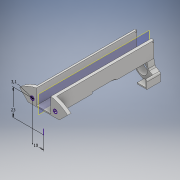
# Autodesk Inventor part: Hull_batt_pillar3
Saved by Autodesk Inventor 2018.2 (Build 222227000, 227)
## iProperties
Created: 2018-05-01
Part Number: Hull_batt_pillar3
Material: Generic
Document SubType Name: Modeling
Designer: suchanek
Density: 1 g/cm^3
Appearance: Default
Author: suchanek
Autodesk Inventor part; units mm, degrees
ref_plane "YZ Plane" through (0, 0, 0) normal (1, 0, 0) x (0, 1, 0)
ref_plane "XZ Plane" through (0, 0, 0) normal (0, 1, 0) x (-1, 0, 0)
ref_plane "XY Plane" through (0, 0, 0) normal (0, 0, 1) x (1, 0, 0)
sketch "Sketch1" plane through (0, 0, 0) normal (0, 1, 0) x (-1, 0, 0)
  arc A0 (21.0006, 25.4554) -> (6.35, 32.3833) centre (0, 0) ccw
  line L0 (0, 0) -> (-23.3345, 23.3345)
  line L1 (0, 0) -> (33, 0) construction
  line L2 (0, 0) -> (0, 8.3369)
  line L3 (-23.3345, 23.3345) -> (-9.1924, 9.1924)
  line L4 (-9.1924, 9.1924) -> (-6.965, 11.4198)
  line L5 (-6.965, 11.4198) -> (-13.7089, 18.1636)
  line L6 (-21.1071, 25.5619) -> (-23.3345, 23.3345)
  line L7 (23.3345, 23.3345) -> (9.1924, 9.1924)
  line L8 (9.1924, 9.1924) -> (6.965, 11.4198)
  line L9 (6.965, 11.4198) -> (13.7089, 18.1636)
  line L10 (21.1071, 25.5619) -> (23.3345, 23.3345)
  line L11 (-6.35, 32.3833) -> (6.35, 32.3833)
  line L12 (6.35, 32.3833) -> (6.35, 19.1636)
  line L13 (6.35, 19.1636) -> (-6.35, 19.1636)
  line L14 (-6.35, 19.1636) -> (-6.35, 32.3833)
  line L15 (13.7089, 18.1636) -> (-13.7089, 18.1636)
  line L16 (-13.7089, 18.1636) -> (-21.1071, 25.5619)
  arc A1 (-6.35, 32.3833) -> (-21.0006, 25.4554) centre (0, 0) ccw
  arc A2 (6.35, 32.3833) -> (-6.35, 32.3833) centre (0, 0) ccw
  line L17 (13.7089, 18.1636) -> (21.1071, 25.5619)
  point P0 (-6.35, 31.3636)
  dimension "d0" = 33
  dimension "d1" = 33
  dimension "d2" = 135
  dimension "d3" = 3.15
  dimension "d4" = 20
  dimension "d5" = 32
  dimension "d7" = 12.2
  dimension "d8" = 12.7
  dimension "d33" = 18.1636
  constraints: 36 end point, 7 point on circle, 6 point on line, 5 parallel, 4 symmetric about line, 3 centre point, 3 horizontal, 2 perpendicular, 1 coincident, 1 equal length, 1 vertical
  measures "d0" radius of A0
  measures "d1" distance of L0.start L0.end
  measures "d2" angle of L1 L0
  measures "d3" distance of L4.end L3.end
  measures "d4" distance between parallel lines of L6 L4
  measures "d5" distance of point (0, 0) point (-6.35, 31.364)
  measures "d7" distance of L13.end point (-6.35, 31.364)
  measures "d8" distance of L12.end L13.end
  measures "d33" distance from line of L0.start L15
extrude "Extrusion1" add sketch "Sketch1" along normal blind 3 contours L17 L15 L16 A1 L14 L13 L12 A0
sketch "Sketch2" plane through (0, 3, 0) normal (0, 1, 0) x (1, 0, 0)
  arc A0 (6.35, -32.3833) -> (21.0006, -25.4554) centre (0, 0) ccw projected
  line L0 (8.35, -31.9261) -> (8.35, -18.1636)
  line L1 (13.7089, -18.1636) -> (-13.7089, -18.1636) projected
  line L2 (-8.35, -18.1636) -> (-8.35, -31.9261)
  arc A1 (-21.0006, -25.4554) -> (-6.35, -32.3833) centre (0, 0) ccw projected
  line L3 (-6.35, -19.1636) -> (6.35, -19.1636) projected
  line L4 (6.35, -32.3833) -> (6.35, -19.1636)
  line L5 (6.35, -19.1636) -> (-6.35, -19.1636)
  line L6 (-6.35, -32.3833) -> (-6.35, -19.1636) projected
  line L7 (-6.35, -19.1636) -> (-6.35, -32.3833)
  dimension "d14" = 2
  constraints: 10 end point, 3 vertical, 2 perpendicular, 2 point on circle, 2 point on line, 1 horizontal alignment
  measures "d14" distance between parallel lines of L6 L2
extrude "Extrusion2" add sketch "Sketch2" along normal blind 85
ref_plane "Work Plane1" through (8.35, 3, 18.1636) normal (-0.7071068, 0, -0.7071068) x (0, 1, 0)
sketch "Sketch4" plane through (8.35, 3, 18.1636) normal (-0.7071068, 0, -0.7071068) x (0, 1, 0)
  circle A0 centre (49, 6.9393) radius 8
  line L0 (85, -9.7316) -> (85, 0) projected
  line L1 (-3, 3.7893) -> (0, 3.7893) projected
  line L2 (49, -1.0607) -> (31, -1.0607)
  line L3 (31, -1.0607) -> (31, 14.9393)
  line L4 (31, 14.9393) -> (49, 14.9393)
  line L5 (49, 14.9393) -> (49, -1.0607)
  point P0 (-3, 6.9393)
  dimension "d19" = 16
  dimension "d20" = 36
  dimension "d21" = 3.15
  dimension "d22" = 18
  dimension "d23" = 16
  constraints: 8 end point, 2 parallel, 2 point on circle, 1 centre point, 1 horizontal, 1 perpendicular
  measures "d19" diameter of A0
  measures "d20" distance from line of L0 A0.centre
  measures "d21" distance from line of L1 A0.centre
  measures "d22" distance of L3.end L4.end
  measures "d23" distance of L2.end L3.end
extrude "Extrusion3" cut sketch "Sketch4" along normal through all both and the other way through all
ref_plane "Work Plane3" through (0, 88, 18.1636) normal (-1, 0, 0) x (0, 0, 1)
mirror "Mirror1" about plane through (0, 88, 18.1636) normal (-1, 0, 0) of "Extrusion3"
sketch "Sketch5" plane through (0, 88, 0) normal (0, 1, 0) x (1, 0, 0)
  line L0 (8.35, -30.3833) -> (-8.35, -30.3833)
  line L1 (-8.35, -30.3833) -> (-8.35, -31.3833)
  line L2 (-8.35, -31.3833) -> (8.35, -31.3833)
  line L3 (8.35, -31.3833) -> (8.35, -30.3833)
  line L4 (8.35, -31.9261) -> (8.35, -18.1636) projected
  arc A0 (6.35, -32.3833) -> (21.0006, -25.4554) centre (0, 0) ccw projected
  dimension "d27" = 16.7
  dimension "d28" = 1
  dimension "d29" = 1
  constraints: 8 end point, 2 parallel, 1 collinear, 1 horizontal, 1 perpendicular
  measures "d27" distance of L2.end L1.end
  measures "d28" distance of L1.end L0.end
  measures "d29" distance from line of A0.start L2
extrude "Extrusion4" cut sketch "Sketch5" against normal blind 1.1
fillet "Fillet1" radius 0.5 4 edges at (7.35, 86.9, 31.3833) (-7.35, 86.9, 31.3833) (-7.35, 86.9, 30.3833) (7.35, 86.9, 30.3833)
sketch "Sketch6" plane through (13.7089, 0, 18.1636) normal (0, 0, -1) x (-1, 0, 0)
  line L0 (8.4589, 16) -> (18.9589, 16)
  line L1 (18.9589, 16) -> (18.9589, 54)
  line L2 (18.9589, 54) -> (8.4589, 54)
  line L3 (8.4589, 54) -> (8.4589, 16)
  line L4 (13.7089, 0) -> (13.7089, 8.6013)
  line L5 (5.3589, 88) -> (22.0589, 88) projected
  dimension "d36" = 10.5
  dimension "d37" = 38
  dimension "d38" = 34
  constraints: 10 end point, 2 parallel, 1 horizontal, 1 perpendicular, 1 vertical, 1 other
  measures "d36" distance of L1.end L2.end
  measures "d37" distance of L0.end L1.end
  measures "d38" distance between parallel lines of L5 L2
extrude "Extrusion5" cut sketch "Sketch6" against normal blind 0.336
sketch "Náčrt7" plane through (0, 0, 0) normal (0, -1, 0) x (1, 0, 0)
  circle A0 centre (-10, 23) radius 1.55
  line L0 (0, 0) -> (0, 4.6263)
  circle A1 centre (10, 23) radius 1.55
  dimension "d39" = 23
  dimension "d40" = 10
  dimension "d41" = 3.1
  constraints: 2 centre point, 2 end point, 1 symmetric about line, 1 vertical, 1 other
  measures "d39" vertical distance of L0.start A0.centre
  measures "d40" horizontal distance of L0.start A0.centre
  measures "d41" diameter of A0
extrude "Vysunutí6" cut sketch "Náčrt7" against normal up to surface (3 mm away)
sketch "Náčrt8" plane through (0, 0, 0) normal (0, -1, 0) x (1, 0, 0)
  line L0 (-10, 20.1132) -> (-12.5, 21.5566)
  line L1 (-12.5, 21.5566) -> (-12.5, 24.4434)
  line L2 (-12.5, 24.4434) -> (-10, 25.8868)
  line L3 (-10, 25.8868) -> (-7.5, 24.4434)
  line L4 (-7.5, 24.4434) -> (-7.5, 21.5566)
  line L5 (-7.5, 21.5566) -> (-10, 20.1132)
  point P0 (0, 0)
  point P1 (-10, 23)
  point P2 (-10, 23)
  dimension "d44" = 2.5
  constraints: 12 end point, 1 coincident, 13 other
  measures "d44" distance from line of L4 point (-10, 23)
extrude "Vysunutí7" cut sketch "Náčrt8" against normal blind 2 from surface at -3
ref_plane "Pracovní rovina4" through (0, 0, 19.1636) normal (-1, 0, 0) x (0, 0, 1)
mirror "Zrcadlit2" about plane through (0, 0, 19.1636) normal (-1, 0, 0) of "Vysunutí7"
sketch "Náčrt9" plane through (13.7089, 0, 18.4996) normal (0, 0, -1) x (-1, 0, 0)
  line L0 (15.4589, 47.589) -> (13.4589, 47.589)
  line L1 (13.4589, 47.589) -> (13.4589, 53.589)
  line L2 (13.4589, 53.589) -> (15.4589, 53.589)
  line L3 (15.4589, 53.589) -> (15.4589, 47.589)
  line L4 (15.4589, 17.089) -> (13.4589, 17.089)
  line L5 (13.4589, 17.089) -> (13.4589, 23.089)
  line L6 (13.4589, 23.089) -> (15.4589, 23.089)
  line L7 (15.4589, 23.089) -> (15.4589, 17.089)
  line L8 (5.3589, 88) -> (22.0589, 88) projected
  line L9 (13.7089, 105.6) -> (13.7089, -17.6) projected
  point P0 (13.7089, 0)
  dimension "d47" = 34.411
  dimension "d48" = 6
  dimension "d49" = 2
  dimension "d50" = 1.75
  dimension "d51" = 6
  dimension "d52" = 2
  dimension "d53" = 30.5
  constraints: 16 end point, 4 parallel, 2 horizontal, 2 perpendicular, 2 point on line
  measures "d47" distance between parallel lines of L2 L8
  measures "d48" distance between parallel lines of L0 L2
  measures "d49" distance between parallel lines of L1 L3
  measures "d50" distance between parallel lines of L9 L3
  measures "d51" distance between parallel lines of L4 L6
  measures "d52" distance of L5.end L6.end
  measures "d53" distance between parallel lines of L6 L2
extrude "Vysunutí8" add sketch "Náčrt9" along normal blind 5.5
sketch "Náčrt10" plane through (0.25, 17.089, 18.4996) normal (1, 0, 0) x (0, 0, -1)
  circle A0 centre (3, 33.5) radius 1.55
  circle A1 centre (3, 3) radius 1.55
  line L0 (0, 30.5) -> (0, 36.5) projected
  line L1 (0, 0) -> (0, 6) projected
  point P0 (18.4996, -17.089)
  dimension "d56" = 3
  dimension "d57" = 3
  dimension "d58" = 3.1
  dimension "d59" = 3.1
  constraints: 2 centre point
  measures "d56" distance from line of A0.centre L0
  measures "d57" distance from line of L1 A1.centre
  measures "d58" diameter of A0
  measures "d59" diameter of A1
extrude "Vysunutí9" cut sketch "Náčrt10" against normal blind 5.5
fillet "Zaoblení2" radius 2 4 edges at (-0.75, 23.089, 12.9996) (-0.75, 17.089, 12.9996) (-0.75, 53.589, 12.9996) (-0.75, 47.589, 12.9996)
sketch "Náčrt11" plane through (0, 88, 0) normal (0, 1, 0) x (1, 0, 0)
  line L0 (-8.35, -30.3833) -> (-6.35, -30.3833) projected
  line L1 (-6.35, -30.3833) -> (-6.35, -19.1636) projected
  line L2 (-6.35, -19.1636) -> (6.35, -19.1636) projected
  line L3 (6.35, -19.1636) -> (6.35, -30.3833) projected
  line L4 (6.35, -30.3833) -> (8.35, -30.3833) projected
  line L5 (8.35, -30.3833) -> (8.35, -18.1636) projected
  line L6 (8.35, -18.1636) -> (-8.35, -18.1636) projected
  line L7 (-8.35, -18.1636) -> (-8.35, -30.3833) projected
  circle A0 centre (3.85, -11.5636) radius 5
  arc A1 (0.9157, -6.3301) -> (-1.9615, -10.0715) centre (3.85, -11.5636) ccw
  line L8 (6.8499, -18.1636) -> (8.35, -18.1636) projected
  line L9 (8.35, -18.1636) -> (9.4474, -13.8894)
  line L10 (-1.9615, -10.0715) -> (-4.0392, -18.1636)
  line L11 (5.25, -18.1636) -> (-5.25, -18.1636) projected
  line L12 (-4.0392, -18.1636) -> (8.35, -18.1636)
  line L13 (5.25, -18.4996) -> (-5.25, -18.4996) projected
  line L14 (5.85, -3.5636) -> (14.35, -3.5636)
  line L15 (14.35, -3.5636) -> (14.35, -9.2762)
  line L16 (13.3206, -11.025) -> (10.414, -12.6381)
  line L17 (5.85, -3.5636) -> (0.9157, -6.3301)
  arc A2 (10.414, -12.6381) -> (9.4474, -13.8894) centre (11.3846, -14.3868) ccw
  arc A3 (13.3206, -11.025) -> (14.35, -9.2762) centre (12.35, -9.2762) ccw
  point P0 (0, 0)
  point P1 (9.6615, -13.0558)
  dimension "d63" = 4.5
  dimension "d64" = 6.6
  dimension "d65" = 10
  dimension "d66" = 12
  dimension "d70" = 8
  dimension "d71" = 2
  dimension "d72" = 10.5
  dimension "d73" = 2
  constraints: 14 end point, 7 tangent, 6 point on circle, 4 centre point, 3 point on line, 2 parallel, 1 coincident, 1 equal radius, 1 horizontal, 1 vertical
  measures "d63" distance from line of A0.centre L5
  measures "d64" distance from line of A0.centre L6
  measures "d65" diameter of A0
  measures "d66" diameter of A1
  measures "d70" distance from line of A0.centre L14
  measures "d71" horizontal distance of L14.start A0.centre
  measures "d72" horizontal distance of L14.end A0.centre
  measures "d73" radius of A2
extrude "Vysunutí10" add sketch "Náčrt11" against normal blind 6 contours L10 A1 L17 L14 L15 A3 L16 A2 L9 L6
fillet "Zaoblení3" radius 2 1 edges at (-4.0392, 85, 18.1636)
sketch "Náčrt12" plane through (0, 82, 0) normal (0, -1, 0) x (1, 0, 0)
  circle A0 centre (3.85, 11.5636) radius 5 projected
  line L0 (9.4474, 13.8894) -> (8.35, 18.1636) projected
  line L1 (-5.5906, 18.1636) -> (8.35, 18.1636) projected
  arc A1 (-3.6534, 16.661) -> (-5.5906, 18.1636) centre (-5.5906, 16.1636) ccw projected
  line L2 (-3.6534, 16.661) -> (-1.9615, 10.0715) projected
  arc A2 (-1.9615, 10.0715) -> (0.9157, 6.3301) centre (3.85, 11.5636) ccw projected
  line L3 (0.9157, 6.3301) -> (5.85, 3.5636) projected
  line L4 (5.85, 3.5636) -> (14.35, 3.5636) projected
  line L5 (14.35, 3.5636) -> (14.35, 9.2762) projected
  arc A3 (14.35, 9.2762) -> (13.3206, 11.025) centre (12.35, 9.2762) ccw projected
  line L6 (13.3206, 11.025) -> (10.414, 12.6381) projected
  arc A4 (9.4474, 13.8894) -> (10.414, 12.6381) centre (11.3846, 14.3868) ccw projected
  line L7 (0.9157, 6.3301) -> (5.85, 3.5636) projected
  line L8 (13.3206, 11.025) -> (10.414, 12.6381) projected
  line L9 (13.35, 4.5636) -> (13.35, 11.0083)
  line L10 (5.85, 4.5636) -> (13.35, 4.5636)
  line L11 (5.85, 3.5636) -> (5.85, 4.5636)
  point P0 (0, 0)
  dimension "d75" = 1
  dimension "d76" = 1
  constraints: 6 end point, 1 horizontal, 1 perpendicular, 1 point on circle, 1 vertical
  measures "d75" distance between parallel lines of L5 L9
  measures "d76" distance between parallel lines of L4 L10
extrude "Vysunutí11" add sketch "Náčrt12" along normal blind 6 contours A3 L5 L4 L11 L10 L9
body "Solid1"
